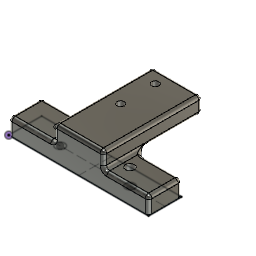
spool_holder_adapter (Autodesk Fusion 360 design; units mm, degrees)
Autodesk Fusion 360 part; units mm, degrees
sketch "Sketch1" plane through (0, 0, 0) normal (0, 0, 1) x (1, 0, 0) in component "spool_holder_adapter"
  line L0 (0, 0) -> (85, 0)
  line L1 (85, 0) -> (85, 20)
  line L2 (85, 20) -> (0, 20)
  line L3 (0, 20) -> (0, 0)
  line L4 (42.5, 20) -> (42.5, 0) construction
  line L5 (0, 10) -> (42.5, 10) construction
  line L6 (85, 10) -> (42.5, 10) construction
  circle A0 centre (21.25, 10) radius 2.7
  circle A1 centre (63.75, 10) radius 2.7
  dimension "d1" = 85
  dimension "d2" = 20
  dimension "d5" = 5.4
  constraint horizontal L0
  constraint vertical L1
  constraint horizontal L2
  constraint vertical L3
  constraint coincident L0.start L3.end
  constraint midpoint L2 L4.start
  constraint midpoint L0 L4.end
  constraint midpoint L3 L5.start
  constraint midpoint L4 L5.end
  constraint midpoint L1 L6.start
  constraint midpoint L5 A0.centre
  constraint symmetric L4 A0 A1
  measures "d1" distance of L0.start L0.end
  measures "d2" distance of L0.start L2.end
  measures "d5" diameter of A0
extrude "Extrude2" add sketch "Sketch1" along normal blind 10 in component "spool_holder_adapter"
sketch "Sketch2" plane through (0, 0, 10) normal (0, 0, 1) x (-1, 0, 0) in component "spool_holder_adapter"
  circle A0 centre (-21.25, -10) radius 2.7
  circle A1 centre (-63.75, -10) radius 2.7
  line L0 (0, -20) -> (0, 0)
  line L1 (0, 0) -> (-85, 0)
  line L2 (-85, 0) -> (-85, -20)
  line L3 (-85, -20) -> (0, -20)
  line L4 (-42.5, -20) -> (-42.5, 0) construction
  line L5 (-42.5, -20) -> (-27.5, -20) construction
  line L6 (-27.5, -20) -> (-57.5, -20)
  line L7 (-57.5, -20) -> (-57.5, -60)
  line L8 (-57.5, -60) -> (-27.5, -60)
  line L9 (-27.5, -60) -> (-27.5, -20)
  line L10 (-27.5, -20) -> (-57.5, -20)
  line L11 (-57.5, -20) -> (-57.5, 0)
  line L12 (-57.5, 0) -> (-27.5, 0)
  line L13 (-27.5, 0) -> (-27.5, -20)
  point P0 (-42.5, -20)
  dimension "d8" = 15
  dimension "d9" = 30
  dimension "d10" = 40
  constraint coincident P0 L4.start
  constraint perpendicular L4 L5
  constraint horizontal L6
  constraint vertical L7
  constraint horizontal L8
  constraint vertical L9
  constraint horizontal L10
  constraint vertical L11
  constraint horizontal L12
  constraint vertical L13
  constraint coincident L1 L11.end
  measures "d8" distance of P0 L5.end
  measures "d9" distance of L5.end L6.end
  measures "d10" distance of L5.end L8.end
extrude "Extrude3" add sketch "Sketch2" along normal blind 10 contours L3 L6 L7 L8 L9 L10 | L1 L3 L6 L10 L11 L12 L13 in component "spool_holder_adapter"
sketch "Sketch3" plane through (0, 0, 20) normal (0, 0, 1) x (-1, 0, 0) in component "spool_holder_adapter"
  line L0 (-57.5, 0) -> (-57.5, -60)
  line L1 (-57.5, -60) -> (-27.5, -60)
  line L2 (-27.5, -60) -> (-27.5, 0)
  line L3 (-27.5, 0) -> (-57.5, 0)
  line L4 (-37.5, -51.5585) -> (-37.5, -30.5585) construction
  circle A0 centre (-37.5, -51.5585) radius 2.2
  circle A1 centre (-37.5, -30.5585) radius 2.2
  line L5 (-37.5, -30.5585) -> (-27.5, -30.5585) construction
  dimension "d13" = 21
  dimension "d14" = 4.4
  dimension "d15" = 4.4
  constraint perpendicular L1 L4
  constraint coincident L4.start A0.centre
  constraint coincident L4.end A1.centre
  constraint coincident L2 L5.end
  constraint perpendicular L2 L5
  measures "d13" distance of L4.start L4.end
  measures "d14" diameter of A0
  measures "d15" diameter of A1
extrude "Extrude4" cut sketch "Sketch3" against normal up to surface (10 mm away) contours A0 | A1 in component "spool_holder_adapter"
sketch "Sketch4" plane through (0, 0, 10) normal (0, 0, -1) x (1, 0, 0) in component "spool_holder_adapter"
  circle A0 centre (37.5, -30.5585) radius 2.2
  circle A1 centre (37.5, -51.5585) radius 2.2
  line L0 (57.5, -20) -> (27.5, -20)
  line L1 (27.5, -20) -> (27.5, -60)
  line L2 (27.5, -60) -> (57.5, -60)
  line L3 (57.5, -60) -> (57.5, -20)
  line L4 (39.462, -55.0443) -> (41.4998, -51.6022)
  line L5 (41.4998, -51.6022) -> (39.5377, -48.1165)
  line L6 (39.5377, -48.1165) -> (35.538, -48.0728)
  line L7 (35.538, -48.0728) -> (33.5002, -51.5149)
  line L8 (33.5002, -51.5149) -> (35.4623, -55.0006)
  line L9 (35.4623, -55.0006) -> (39.462, -55.0443)
  line L10 (37.5, -30.5585) -> (37.5, -51.5585) construction
  line L11 (37.5, -51.5585) -> (37.5, -41.0585) construction
  line L12 (37.5, -41.0585) -> (22.4999, -41.0585) construction
  line L13 (39.5377, -34.0006) -> (35.538, -34.0443)
  line L14 (41.4998, -30.5149) -> (39.5377, -34.0006)
  line L15 (39.462, -27.0728) -> (41.4998, -30.5149)
  line L16 (35.4623, -27.1165) -> (39.462, -27.0728)
  line L17 (33.5002, -30.6022) -> (35.4623, -27.1165)
  line L18 (35.538, -34.0443) -> (33.5002, -30.6022)
  point P0 (37.5, -51.5585)
  dimension "d18" = 4
  constraint coincident P0 A1.centre
  constraint coincident A0.centre L10.start
  constraint midpoint L10 L11.end
  constraint horizontal L12
  constraint symmetric L4.start L12 L15.start
  constraint symmetric L4.end L12 L14.start
  constraint symmetric L5.end L12 L13.start
  constraint symmetric L6.end L12 L13.end
  constraint symmetric L7.end L12 L17.start
  constraint symmetric L8.end L12 L16.start
  measures "d18" distance of L4.start P0
extrude "Extrude5" cut sketch "Sketch4" against normal blind 3.2 contours L4 L5 L6 L7 L8 L9 | L13 L14 L15 L16 L17 L18 in component "spool_holder_adapter"
fillet "Fillet1" radius 7 1 edges at (42.5, 20, 10) in component "spool_holder_adapter"
fillet "Fillet2" radius 5 1 edges at (57.5, 20, 6.5) in component "spool_holder_adapter"
fillet "Fillet3" radius 5 1 edges at (27.5, 20, 6.5) in component "spool_holder_adapter"
fillet "Fillet4" radius 2 1 edges at (57.5, 12.5, 10) in component "spool_holder_adapter"
fillet "Fillet5" radius 2 1 edges at (27.5, 12.5, 10) in component "spool_holder_adapter"
fillet "Fillet6" radius 2 11 edges at (0, 10, 10) (27.5, 30, 20) (57.5, 30, 20) (85, 10, 10) (85, 20, 5) (73.75, 20, 10) (60.9189, 20.2566, 10) (57.9939, 22.8331, 10.684) (27.0061, 22.8331, 10.684) (24.0811, 20.2566, 10) (11.25, 20, 10) in component "spool_holder_adapter"
fillet "Fillet7" radius 2 15 edges at (0, 20, 4) (0.5858, 19.4142, 9.4142) (0, 0, 4) (0.5858, 0, 9.4142) (13.75, 0, 10) (26.9142, 0, 10.5858) (27.5, 0, 15) (28.0858, 0, 19.4142) (42.5, 0, 20) (56.9142, 0, 19.4142) (57.5, 0, 15) (58.0858, 0, 10.5858) (71.25, 0, 10) (84.4142, 0, 9.4142) (85, 0, 4) in component "spool_holder_adapter"
fillet "Fillet8" radius 2 12 edges at (27.5, 43.5, 10) (27.5, 25.9894, 9.9267) (25.7491, 21.2005, 6.9185) (42.5, 60, 10) (59.2509, 21.2005, 6.9185) (57.5, 25.9894, 9.9267) (57.5, 43.5, 10) (57.5, 60, 14) (56.9142, 60, 19.4142) (42.5, 60, 20) (28.0858, 60, 19.4142) (27.5, 60, 14) in component "spool_holder_adapter"
component "spool_holder_adapter" placed x (1, 0, 0) y (0, 1, 0) z (0, 0, 1) at (0, 0, 0)
